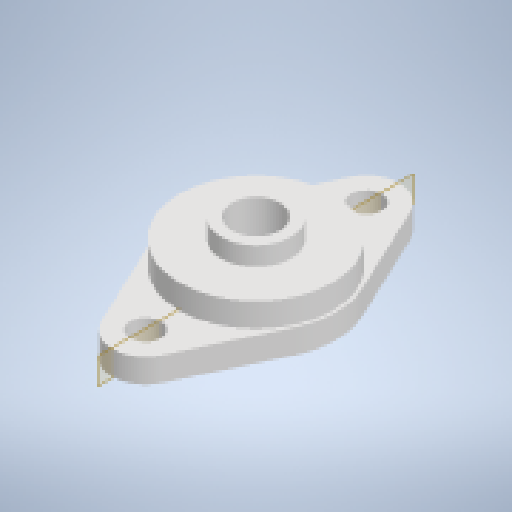
# Autodesk Inventor part: Bearing
Saved by Autodesk Inventor 2025 (Build 290162000, 162)
## iProperties
Created: 2025-07-18
Part Number: Bearing
Material: Generic
Document SubType Name: Modeling
Designer: yshis
Density: 1 g/cm^3
Appearance: Default
Author: yshis
Autodesk Inventor part; units mm, degrees
ref_plane "YZ Plane" through (0, 0, 0) normal (1, 0, 0) x (0, 1, 0)
ref_plane "XZ Plane" through (0, 0, 0) normal (0, 1, 0) x (-1, 0, 0)
ref_plane "XY Plane" through (0, 0, 0) normal (0, 0, 1) x (1, 0, 0)
sketch "Sketch1" plane through (0, 0, 0) normal (0, 1, 0) x (-1, 0, 0)
  circle A0 centre (0, -18.35) radius 2.5
  circle A1 centre (0, 18.35) radius 2.5
  circle A2 centre (0, 0) radius 4
  circle A3 centre (0, 0) radius 5.8
  circle A4 centre (0, 0) radius 12.75
  line L0 (4.9784, -20.6879) -> (12.0386, -5.6534)
  line L1 (-4.9784, -20.6879) -> (-12.0386, -5.6534)
  line L2 (4.9784, 20.6879) -> (12.0386, 5.6534)
  line L3 (-4.9784, 20.6879) -> (-12.0386, 5.6534)
  arc A5 (-4.9784, -20.6879) -> (4.9784, -20.6879) centre (0, -18.35) ccw
  arc A6 (4.9784, 20.6879) -> (-4.9784, 20.6879) centre (0, 18.35) ccw
  arc A7 (-12.0386, 5.6534) -> (-12.0386, -5.6534) centre (0, 0) ccw
  arc A8 (12.0386, -5.6534) -> (12.0386, 5.6534) centre (0, 0) ccw
  dimension "d2" = 18.35
  dimension "d4" = 18.35
  dimension "d5" = 5
  dimension "d6" = 5
  dimension "d7" = 8
  dimension "d8" = 11.6
  dimension "d9" = 25.5
  dimension "d10" = 0
  dimension "d12" = 0
  constraints: 9 centre point, 8 end point, 8 point on circle, 8 tangent, 6 coincident
  measures "d2" distance of point (0, 0) A5.centre
  measures "d4" distance of A6.centre point (0, 0)
  measures "d5" diameter of A0
  measures "d6" diameter of A1
  measures "d7" diameter of A2
  measures "d8" diameter of A3
  measures "d9" diameter of A4
  measures "d10" horizontal distance of point (0, 0) A5.centre
  measures "d12" horizontal distance of A6.centre point (0, 0)
extrude "Extrusion1" add sketch "Sketch1" along normal blind 11.1 contours A3
sketch "Sketch2" plane through (0, 0, 0) normal (0, -1, 0) x (1, 0, 0)
  circle A0 centre (0, -18.35) radius 2.5
  circle A1 centre (0, 18.35) radius 2.5
  circle A2 centre (0, 0) radius 4
  circle A3 centre (0, 0) radius 5.8
  circle A4 centre (0, 0) radius 12.75
  line L0 (4.9784, -20.6879) -> (12.0386, -5.6534)
  line L1 (-4.9784, -20.6879) -> (-12.0386, -5.6534)
  line L2 (4.9784, 20.6879) -> (12.0386, 5.6534)
  line L3 (-4.9784, 20.6879) -> (-12.0386, 5.6534)
  arc A5 (-4.9784, -20.6879) -> (4.9784, -20.6879) centre (0, -18.35) ccw
  arc A6 (4.9784, 20.6879) -> (-4.9784, 20.6879) centre (0, 18.35) ccw
  arc A7 (-12.0386, 5.6534) -> (-12.0386, -5.6534) centre (0, 0) ccw
  arc A8 (12.0386, -5.6534) -> (12.0386, 5.6534) centre (0, 0) ccw
  dimension "d15" = 18.35
  dimension "d16" = 18.35
  dimension "d17" = 5
  dimension "d18" = 5
  dimension "d19" = 8
  dimension "d20" = 11.6
  dimension "d21" = 25.5
  dimension "d22" = 0
  dimension "d23" = 0
  dimension "d24" = 0
  dimension "d25" = 0
  constraints: 9 centre point, 8 end point, 8 point on circle, 8 tangent, 6 coincident
  measures "d15" distance of point (0, 0) A5.centre
  measures "d16" distance of A6.centre point (0, 0)
  measures "d17" diameter of A0
  measures "d18" diameter of A1
  measures "d19" diameter of A2
  measures "d20" diameter of A3
  measures "d21" diameter of A4
  measures "d22" horizontal distance of point (0, 0) A5.centre
  measures "d23" horizontal distance of A6.centre point (0, 0)
  measures "d24" distance of point (0, 0) point (0, 0)
  measures "d25" distance of point (0, 0) point (0, 0)
extrude "Extrusion2" add sketch "Sketch2" against normal blind 8 contours A4
sketch "Sketch3" plane through (0, 0, 0) normal (0, -1, 0) x (1, 0, 0)
  circle A0 centre (0, -18.35) radius 2.5
  circle A1 centre (0, 18.35) radius 2.5
  circle A2 centre (0, 0) radius 4
  line L0 (4.9784, -20.6879) -> (12.0386, -5.6534)
  line L1 (-4.9784, -20.6879) -> (-12.0386, -5.6534)
  line L2 (4.9784, 20.6879) -> (12.0386, 5.6534)
  line L3 (-4.9784, 20.6879) -> (-12.0386, 5.6534)
  arc A3 (-4.9784, -20.6879) -> (4.9784, -20.6879) centre (0, -18.35) ccw
  arc A4 (4.9784, 20.6879) -> (-4.9784, 20.6879) centre (0, 18.35) ccw
  arc A5 (-12.0386, 5.6534) -> (-12.0386, -5.6534) centre (0, 0) ccw
  arc A6 (12.0386, -5.6534) -> (12.0386, 5.6534) centre (0, 0) ccw
  dimension "d28" = 18.35
  dimension "d29" = 18.35
  dimension "d30" = 5
  dimension "d31" = 5
  dimension "d32" = 8
  dimension "d35" = 0
  dimension "d36" = 0
  dimension "d37" = 0
  dimension "d38" = 0
  constraints: 8 end point, 8 point on circle, 8 tangent, 7 centre point, 4 coincident
  measures "d28" distance of point (0, 0) A3.centre
  measures "d29" distance of A4.centre point (0, 0)
  measures "d30" diameter of A0
  measures "d31" diameter of A1
  measures "d32" diameter of A2
  measures "d35" horizontal distance of point (0, 0) A3.centre
  measures "d36" horizontal distance of A4.centre point (0, 0)
  measures "d37" distance of point (0, 0) point (0, 0)
  measures "d38" distance of point (0, 0) point (0, 0)
extrude "Extrusion3" add sketch "Sketch3" against normal blind 4
ref_plane "Work Plane1" through (0, 4, 23.85) normal (1, 0, 0) x (0, -1, 0)
equation "\"d4\" = d2"
equation "\"d16\" = d15"
equation "\"d29\" = d28"
body "Solid1"
